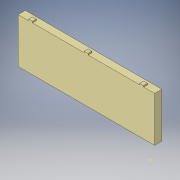
# Autodesk Inventor part: Breadboard
Saved by Autodesk Inventor 2016 (Build 200138000, 138)
## iProperties
Created: 2016-10-04
Part Number: Breadboard
Material: Generic
Document SubType Name: Modeling
Designer: desirw
Density: 1 g/cm^3
Appearance: Default
Author: desirw
Autodesk Inventor part; units mm, degrees
ref_plane "YZ Plane" through (0, 0, 0) normal (1, 0, 0) x (0, 1, 0)
ref_plane "XZ Plane" through (0, 0, 0) normal (0, 1, 0) x (-1, 0, 0)
ref_plane "XY Plane" through (0, 0, 0) normal (0, 0, 1) x (1, 0, 0)
sketch "Sketch1" plane through (0, 0, 0) normal (0, 0, 1) x (1, 0, 0)
  line L0 (-150.6651, 27.0609) -> (14.4349, 27.0609)
  line L1 (14.4349, 27.0609) -> (14.4349, 81.4169)
  line L2 (14.4349, 81.4169) -> (-150.6651, 81.4169)
  line L3 (-150.6651, 81.4169) -> (-150.6651, 27.0609)
  point P0 (0, 0)
  dimension "d0" = 165.1
  dimension "d1" = 54.356
  constraints: 8 end point, 2 parallel, 1 horizontal, 1 perpendicular
  measures "d0" distance of L2.end L1.end
  measures "d1" distance of L1.end L0.end
extrude "Extrusion1" add sketch "Sketch1" along normal blind 8.763
sketch "Sketch2" plane through (-150.6651, 81.4169, 0) normal (0, 1, 0) x (1, 0, 0)
  line L0 (0, -8.763) -> (165.1, -8.763) projected
  line L1 (12.7, -8.763) -> (17.399, -8.763)
  line L2 (17.399, -8.763) -> (17.399, -4.064)
  line L3 (17.399, -4.064) -> (12.7, -4.064)
  line L4 (12.7, -4.064) -> (12.7, -8.763)
  line L5 (0, 0) -> (0, -8.763) projected
  line L6 (79.883, -4.064) -> (79.883, -8.763)
  line L7 (84.582, -4.064) -> (79.883, -4.064)
  line L8 (84.582, -8.763) -> (84.582, -4.064)
  line L9 (79.883, -8.763) -> (84.582, -8.763)
  line L10 (147.066, -4.064) -> (147.066, -8.763)
  line L11 (151.765, -4.064) -> (147.066, -4.064)
  line L12 (151.765, -8.763) -> (151.765, -4.064)
  line L13 (147.066, -8.763) -> (151.765, -8.763)
  point P0 (150.6651, 0)
  dimension "d4" = 4.699
  dimension "d5" = 4.699
  dimension "d6" = 12.7
  dimension "d9" = 67.183
  constraints: 24 end point, 2 horizontal, 2 parallel, 1 perpendicular, 1 point on line, 16 other
  measures "d4" distance of L3.end L2.end
  measures "d5" distance of L2.end L1.end
  measures "d6" distance between parallel lines of L5 L4
  measures "d9" distance of L3.end L6.start
extrude "Extrusion2" add sketch "Sketch2" along normal blind 1.651
sketch "Sketch3" plane through (0, 0, 0) normal (0, 0, -1) x (-1, 0, 0)
  line L0 (57.8264, 56.7985) -> (80.4764, 56.7985) construction
  line L1 (80.4764, 56.7985) -> (80.4764, 50.7025) construction
  line L2 (80.4764, 50.7025) -> (57.8264, 50.7025) construction
  line L3 (57.8264, 50.7025) -> (57.8264, 56.7985) construction
  point P0 (0, 0)
  constraints: 2 other
body "Solid1"
